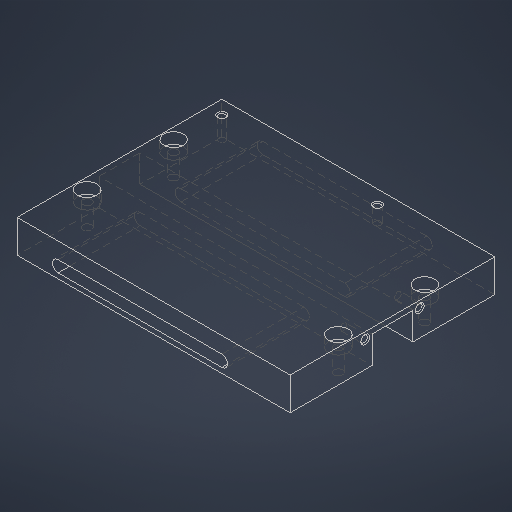
# Autodesk Inventor part: blat
Saved by Autodesk Inventor 2026.1 (Build 301233020, 233B)
## iProperties
Created: 2025-11-04
Part Number: blat
Material: Stainless Steel, Austenitic
Document SubType Name: Modeling
Designer: Jan
Density: 8 g/cm^3
Appearance: Semi-Polished
Author: Jan
Autodesk Inventor part; units mm, degrees
ref_plane "YZ Plane" through (0, 0, 0) normal (1, 0, 0) x (0, 1, 0)
ref_plane "XZ Plane" through (0, 0, 0) normal (0, 1, 0) x (-1, 0, 0)
ref_plane "XY Plane" through (0, 0, 0) normal (0, 0, 1) x (1, 0, 0)
sketch "Sketch1" plane through (0, 0, 0) normal (0, 1, 0) x (-1, 0, 0)
  line L0 (0, 0) -> (100, 0)
  line L1 (100, 0) -> (100, -75)
  line L2 (100, -75) -> (0, -75)
  line L3 (0, -75) -> (0, 0)
  line L4 (100, -75) -> (100, 0)
  dimension "d0" = 100
  dimension "d1" = 75
  constraints: 10 end point, 2 parallel, 1 horizontal, 1 perpendicular
  measures "d0" distance of L1.end L2.end
  measures "d1" distance of L0.end L1.end
extrude "Extrusion1" add sketch "Sketch1" along normal blind 12
sketch "Sketch2" plane through (0, 0, 0) normal (1, 0, 0) x (0, 0, -1)
  line L0 (0, 0) -> (75, 0) projected
  line L1 (30, 0) -> (45, 0)
  line L2 (45, 0) -> (45, 10)
  line L3 (45, 10) -> (30, 10)
  line L4 (30, 10) -> (30, 0)
  line L5 (75, 0) -> (75, 12) projected
  line L6 (0, 0) -> (0, 12) projected
  point P0 (0, 6)
  point P1 (30, 5)
  point P2 (45, 0)
  dimension "d12" = 15
  dimension "d13" = 75
  dimension "d14" = 30
  dimension "d15" = 10
  constraints: 8 end point, 2 midpoint, 2 parallel, 1 horizontal, 1 perpendicular, 1 point on line
  measures "d12" distance of L3.end L2.end
  measures "d13" distance from line of L5 point (0, 6)
  measures "d14" distance from line of point (30, 5) L6
  measures "d15" distance of L1.start L3.end
extrude "Extrusion2" cut sketch "Sketch2" against normal through all
sketch "Sketch3" plane through (-100, 0, 0) normal (0, 0, 1) x (1, 0, 0)
  line L0 (0, 0) -> (0, 12) projected
  line L1 (15, 4) -> (75, 4) construction
  line L2 (15, 1.9) -> (75, 1.9)
  line L3 (75, 6.1) -> (15, 6.1)
  arc A0 (15, 6.1) -> (15, 1.9) centre (15, 4) ccw
  arc A1 (75, 1.9) -> (75, 6.1) centre (75, 4) ccw
  line L4 (0, 0) -> (100, 0) projected
  line L5 (0, 12) -> (100, 12) projected
  point P0 (0, 6)
  point P1 (45, 4)
  point P2 (0, 6)
  dimension "d20" = 4.2
  dimension "d21" = 15
  dimension "d22" = 4
  dimension "d23" = 12
  dimension "d60" = 60
  constraints: 8 end point, 4 point on circle, 4 tangent, 3 midpoint, 2 centre point, 1 horizontal, 1 parallel
  measures "d20" diameter of A1
  measures "d21" horizontal distance of point (0, 6) L1.start
  measures "d22" distance from line of L4 L1.start
  measures "d23" distance between parallel lines of L4 L5
  measures "d60" distance of L1.end L1.start
extrude "Extrusion3" cut sketch "Sketch3" against normal through all
sketch "Sketch4" plane through (0, 0, -75) normal (1, 0, 0) x (0, 0, -1)
  circle A0 centre (-27.5, 9.5) radius 1.5
  line L0 (-30, 0) -> (0, 0) projected
  line L1 (-30, 10) -> (-30, 0) projected
  line L2 (-30, 0) -> (-45, 0) construction
  line L3 (-45, 0) -> (-37.5, 0) construction
  line L4 (-37.5, 0) -> (-37.5, -2.8944) construction
  circle A1 centre (-47.5, 9.5) radius 1.5
  line L5 (-75, 12) -> (0, 12) projected
  point P0 (-75, 0)
  dimension "d26" = 3
  dimension "d29" = 2.5
  dimension "d30" = 2.5
  constraints: 6 end point, 2 centre point, 1 midpoint, 1 symmetric about line, 1 vertical, 1 other
  measures "d26" diameter of A0
  measures "d29" distance from line of L1 A0.centre
  measures "d30" distance from line of A0.centre L5
hole "Hole1" at (0, 9.5, -27.5) at (0, 9.5, -47.5) direction (-1, 0, 0) diameter 2.459 depth 8 tip angle 118 thread size "M3x0.5" class "6H" standard "ISO Metric profile"
chamfer "Chamfer2" distance 0.4 angle 45 2 edges at (0, 9.5, -46.2705) (0, 9.5, -26.2705)
sketch "Sketch6" plane through (0, 12, 0) normal (0, 1, 0) x (1, 0, 0)
  circle A0 centre (-96, 21.66) radius 1
  line L0 (-100, 0) -> (0, 0) projected
  line L1 (-100, 75) -> (-100, 0) projected
  line L2 (-100, 37.5) -> (-44.6159, 37.5) construction
  line L3 (-50, 0) -> (-50, 87.3463) construction
  circle A1 centre (-4, 21.66) radius 1
  circle A2 centre (-96, 53.34) radius 1
  circle A3 centre (-4, 53.34) radius 1
  point P0 (-96, 21.66)
  point P1 (-4, 21.66)
  point P2 (-4, 21.66)
  point P3 (-96, 53.34)
  point P4 (-4, 53.34)
  point P5 (-4, 53.34)
  dimension "d49" = 2
  dimension "d50" = 21.66
  dimension "d52" = 4
  constraints: 7 symmetric about line, 4 centre point, 4 end point, 2 midpoint, 1 horizontal, 1 vertical, 3 other
  measures "d49" diameter of A0
  measures "d50" distance from line of L0 A0.centre
  measures "d52" distance from line of L1 A0.centre
hole "Hole3" at (-96, 12, -21.66) at (-96, 12, -53.34) at (-4, 12, -53.34) at (-4, 12, -21.66) direction (0, -1, 0) diameter 3.2 depth 13 tip angle 118 counterbore diameter 7.2 counterbore depth 4
sketch "Sketch8" plane through (0, 12, 0) normal (0, 1, 0) x (1, 0, 0)
  circle A0 centre (-95, 70) radius 2
  line L0 (0, 0) -> (0, 75) construction
  line L1 (0, 37.5) -> (-49.0535, 37.5) construction
  line L2 (-100, 75) -> (-100, 0) projected
  line L3 (0, 75) -> (-100, 75) projected
  line L4 (-66.5, 46.7026) -> (-66.5, 27.8899) construction
  circle A1 centre (-38, 70) radius 2
  point P0 (-38, 70)
  dimension "d61" = 4
  dimension "d75" = 5
  dimension "d76" = 57
  dimension "d77" = 5
  constraints: 4 end point, 2 centre point, 2 symmetric about line, 1 horizontal, 1 midpoint, 1 vertical, 1 other
  measures "d61" diameter of A0
  measures "d75" distance from line of L3 A0.centre
  measures "d76" distance of point (-38, 70) A0.centre
  measures "d77" distance from line of L2 A0.centre
hole "Hole4" at (-95, 12, -70) at (-38, 12, -70) direction (0, -1, 0) diameter 2.459 depth 8 tip angle 118 thread size "M3x0.5" class "6H" standard "ISO Metric profile"
chamfer "Chamfer3" distance 0.4 angle 45 2 edges at (-95, 12, -71.2295) (-38, 12, -71.2295)
equation "\"d22\" = 0.333333 * d23"
equation "\"d29\" = d28"
equation "\"d28\" = 2.5"
body "Solid1"
